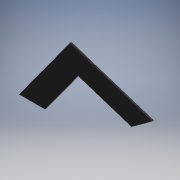
# Autodesk Inventor part: 上部端盖
Saved by Autodesk Inventor 2018 (Build 220112000, 112)
## iProperties
Created: 2021-02-25
Part Number: 上部端盖
Material: 橡胶
Document SubType Name: Modeling
Designer: OHHHHHHHHHH
Density: 0.93 g/cm^3
Appearance: 橡胶 - 黑色
Author: OHHHHHHHHHH
## iProperties of the stored document 上部端盖1_3D 打印.ipt
Created: 2021-03-03
Part Number: 上部端盖1_3D 打印
Material: 常规
Document SubType Name: Modeling
Designer: OHHHHHHHHHH
Density: 1 g/cm^3
Appearance: 默认
Author: OHHHHHHHHHH
Autodesk Inventor part; units mm, degrees
ref_plane "YZ Plane" through (0, 0, 0) normal (1, 0, 0) x (0, 1, 0)
ref_plane "XZ Plane" through (0, 0, 0) normal (0, 1, 0) x (-1, 0, 0)
ref_plane "XY Plane" through (0, 0, 0) normal (0, 0, 1) x (1, 0, 0)
sketch "草图1" plane through (0, 0, 0) normal (0, 1, 0) x (-1, 0, 0)
  line L0 (68.3073, 0) -> (21.1081, -64.9641)
  line L1 (21.1081, -64.9641) -> (-55.2617, -40.15)
  line L2 (-55.2617, -40.15) -> (-55.2617, 40.15)
  line L3 (-55.2617, 40.15) -> (21.1081, 64.9641)
  line L4 (21.1081, 64.9641) -> (68.3073, 0)
  line L5 (105.0554, 0) -> (32.4639, -99.9136)
  line L6 (32.4639, -99.9136) -> (-84.9916, -61.75)
  line L7 (-84.9916, -61.75) -> (-84.9916, 61.75)
  line L8 (-84.9916, 61.75) -> (32.4639, 99.9136)
  line L9 (32.4639, 99.9136) -> (105.0554, 0)
  point P0 (0, 0)
  point P1 (0, 0)
  point P2 (0, 0)
  dimension "d0" = 80.3
  dimension "d1" = 123.5
  constraints: 20 end point, 2 coincident, 22 other
  measures "d0" distance of L1.end L2.end
  measures "d1" distance of L6.end L7.end
extrude "拉伸1" add sketch "草图1" along normal blind 2
sketch "草图2" plane through (0, 2, 0) normal (0, 1, 0) x (1, 0, 0)
  line L0 (-21.1081, 64.9641) -> (55.2617, 40.15) projected
  line L1 (55.2617, 40.15) -> (55.2617, -40.15) projected
  line L2 (55.2617, -40.15) -> (-21.1081, -64.9641) projected
  line L3 (-21.1081, -64.9641) -> (-68.3073, 0) projected
  line L4 (-68.3073, 0) -> (-21.1081, 64.9641) projected
  line L5 (-32.4639, 99.9136) -> (-105.0554, 0) projected
  line L6 (-105.0554, 0) -> (-32.4639, -99.9136) projected
  line L7 (-32.4639, -99.9136) -> (84.9916, -61.75) projected
  line L8 (84.9916, -61.75) -> (84.9916, 61.75) projected
  line L9 (84.9916, 61.75) -> (-32.4639, 99.9136) projected
  line L10 (58.7617, 42.6929) -> (-22.445, 69.0786)
  line L11 (-22.445, 69.0786) -> (-72.6335, 0)
  line L12 (-72.6335, 0) -> (-22.445, -69.0786)
  line L13 (-22.445, -69.0786) -> (58.7617, -42.6929)
  line L14 (58.7617, -42.6929) -> (58.7617, 42.6929)
  line L15 (-23.2089, 71.4297) -> (60.7617, 44.146)
  line L16 (60.7617, 44.146) -> (60.7617, -44.146)
  line L17 (60.7617, -44.146) -> (-23.2089, -71.4297)
  line L18 (-23.2089, -71.4297) -> (-75.1056, 0)
  line L19 (-75.1056, 0) -> (-23.2089, 71.4297)
  point P0 (0, 0)
  dimension "d4" = 3.5
  dimension "d5" = 2
  constraints: 20 end point, 8 other
  measures "d4" distance between parallel lines of L10 L0
  measures "d5" distance between parallel lines of L15 L10
extrude "拉伸2" add sketch "草图2" along normal blind 10 contours L15 L16 L17 L18 L19
sketch "草图3" plane through (0, 0, 0) normal (0, -1, 0) x (1, 0, 0)
  line L0 (-9.4145, -72.1274) -> (53.3776, -50.8644)
  line L1 (53.3776, -50.8644) -> (57.7542, -63.7889)
  line L2 (57.7542, -63.7889) -> (-5.038, -85.0518)
  line L3 (-5.038, -85.0518) -> (-9.4145, -72.1274)
  point P0 (0, 0)
  constraints: 8 end point, 3 perpendicular
extrude "拉伸3" cut sketch "草图3" against normal blind 10
sketch "草图4" plane through (0, 0, 0) normal (0, -1, 0) x (1, 0, 0)
  line L0 (-105.0554, 0) -> (-32.4639, -99.9136) projected
  line L1 (-105.0554, 0) -> (0, 0)
  line L2 (0, 0) -> (99.3977, 72.2167)
  line L3 (99.3977, 72.2167) -> (-62.0091, 125.592)
  line L4 (-62.0091, 125.592) -> (-127.7953, 9.1282)
  line L5 (-127.7953, 9.1282) -> (-105.0554, 0)
  constraints: 10 end point, 1 horizontal, 1 perpendicular
extrude "拉伸4" cut sketch "草图4" against normal blind 16.75 keep common part
